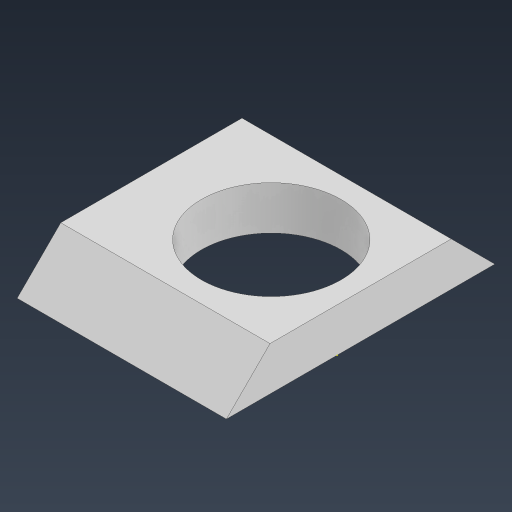
# Autodesk Inventor part: bearing_bed_arm2_tight
Saved by Autodesk Inventor 2024 (Build 280153000, 153)
## iProperties
Created: 2024-10-09
Part Number: bearing_bed_arm2_tight
Material: Generic
Document SubType Name: Modeling
Designer: Piter
Density: 1 g/cm^3
Appearance: Default
Author: Piter
Autodesk Inventor part; units mm, degrees
ref_plane "YZ Plane" through (0, 0, 0) normal (1, 0, 0) x (0, 1, 0)
ref_plane "XZ Plane" through (0, 0, 0) normal (0, 1, 0) x (-1, 0, 0)
ref_plane "XY Plane" through (0, 0, 0) normal (0, 0, 1) x (1, 0, 0)
sketch "Sketch1" plane through (0, 0, 0) normal (0, 1, 0) x (-1, 0, 0)
  line L0 (4.5242, 7.5266) -> (-15.9758, 7.5266)
  line L1 (-15.9758, 7.5266) -> (-15.9758, -12.9734)
  line L2 (-15.9758, -12.9734) -> (4.5242, -12.9734)
  line L3 (4.5242, -12.9734) -> (4.5242, 7.5266)
  circle A0 centre (-5.7258, -2.7234) radius 8
  point P0 (0, 0)
  dimension "d0" = 20.5
  dimension "d1" = 20.5
  dimension "d2" = 16
  constraints: 8 end point, 2 parallel, 1 centre point, 1 horizontal, 1 perpendicular
  measures "d0" distance of L2.end L1.end
  measures "d1" distance of L1.end L0.end
  measures "d2" diameter of A0
extrude "Extrusion1" add sketch "Sketch1" along normal blind 5
sketch "Sketch2" plane through (-4.5242, 0, -12.9734) normal (-1, 0, 0) x (0, 0, 1)
  line L0 (20.5, 0) -> (25.5, 0)
  line L1 (20.5, 0) -> (20.5, 5) projected
  line L2 (25.5, 0) -> (20.5, 5)
  line L3 (0, 0) -> (-5, 0)
  line L4 (-5, 0) -> (0, 5)
  line L5 (0, 0) -> (0, 5) projected
  line L6 (0, 5) -> (0, 0)
  point P0 (12.9734, 0)
  dimension "d6" = 5
  dimension "d7" = 5
  constraints: 10 end point, 2 horizontal, 1 vertical
  measures "d6" distance of L0.start L0.end
  measures "d7" distance of L3.start L3.end
extrude "Extrusion2" add sketch "Sketch2" against normal up to surface (20.5 mm away)
sketch "Sketch3" plane through (15.9758, 0, 12.5266) normal (1, 0, 0) x (0, 0, -1)
  point P0 (12.5266, 0)
sketch "Sketch4" plane through (-4.5242, 0, -17.9734) normal (-1, 0, 0) x (0, 0, 1)
  line L0 (0, 0) -> (30.5, 0) projected
  line L1 (30.5, 0) -> (25.5, 5) projected
  line L2 (5, 5) -> (25.5, 5) projected
  line L3 (5, 5) -> (0, 0) projected
  point P0 (17.9734, 0)
extrude "Extrusion3" add sketch "Sketch4" along normal blind 3.5
sketch "Sketch5" plane through (15.9758, 0, 12.5266) normal (1, 0, 0) x (0, 0, -1)
  line L0 (0, 0) -> (30.5, 0) projected
  line L1 (25.5, 5) -> (30.5, 0) projected
  line L2 (5, 5) -> (25.5, 5) projected
  line L3 (0, 0) -> (5, 5) projected
  line L4 (4.9586, 5.1) -> (25.5414, 5.1)
  line L5 (25.5414, 5.1) -> (30.7414, -0.1)
  line L6 (30.7414, -0.1) -> (-0.2414, -0.1)
  line L7 (-0.2414, -0.1) -> (4.9586, 5.1)
  line L8 (25.5, 5) -> (25.6414, 5)
  line L9 (30.5, 0) -> (30.6414, 0)
  line L10 (0, 0) -> (-0.1414, 0)
  line L11 (5, 5) -> (4.8586, 5)
  point P0 (12.5266, 0)
  dimension "d12" = 0.1
  constraints: 16 end point, 5 point on line, 2 horizontal, 1 parallel, 3 other
  measures "d12" distance between parallel lines of L3 L7
extrude "Extrusion4" add sketch "Sketch5" against normal up to surface (24 mm away) contours L10 L7 L11 L3 | L1 L8 L5 L9
body "Solid1"
